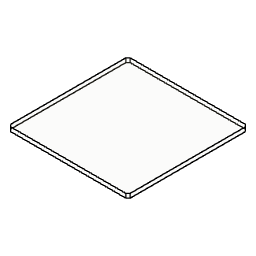
Generic Single Pad Assembly v8 (Autodesk Fusion 360 archive; units mm, degrees)
design "Polycarbonate Top"
Autodesk Fusion 360 part; units mm, degrees
sketch "Sketch1" plane through (0, 0, 0) normal (0, 0, 1) x (1, 0, 0)
  line L0 (132.5, 137.5) -> (-132.5, 137.5)
  line L1 (-137.5, 132.5) -> (-137.5, -132.5)
  line L2 (-132.5, -137.5) -> (132.5, -137.5)
  line L3 (137.5, -132.5) -> (137.5, 132.5)
  line L4 (135, 135) -> (-137.5, -137.5) construction
  line L5 (-137.5, 137.5) -> (135, -135) construction
  line L6 (137.5, 132.5) -> (132.5, 137.5)
  line L7 (-137.5, -132.5) -> (-132.5, -137.5)
  line L8 (-132.5, 137.5) -> (-137.5, 132.5)
  line L9 (137.5, -132.5) -> (132.5, -137.5)
  dimension "d2" = 275
  dimension "d5" = 5
  dimension "d6" = 5
  dimension "d7" = 5
  dimension "d8" = 5
  dimension "d9" = 5
  dimension "d10" = 5
  constraint horizontal L0
  constraint perpendicular L0 L1
  constraint parallel L0 L2
  constraint parallel L1 L3
  constraint coincident L4 origin
  constraint coincident L5 origin
  constraint coincident L3.end L6.start
  constraint coincident L0.start L6.end
  constraint coincident L6 L4.start
  constraint coincident L1.end L7.start
  constraint coincident L2.start L7.end
  constraint perpendicular L4 L7
  constraint coincident L0.end L8.start
  constraint coincident L1.start L8.end
  constraint coincident L3.start L9.start
  constraint coincident L2.end L9.end
  constraint coincident L9 L5.end
  measures "d2" distance of L5.start L4.end
  measures "d5" distance of L2 L3.start
  measures "d6" distance of L3 L2.end
  measures "d7" distance of L1 L0.end
  measures "d8" distance of L0 L1.start
  measures "d9" distance of L2 L1.end
  measures "d10" distance of L1 L2.start
extrude "Extrude1" add sketch "Sketch1" along normal blind 9.525
equation "d11 = 3 / 8 * in"

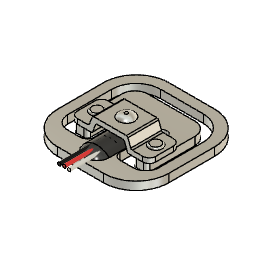
design "SparkFun Generic Load Cell"
Autodesk Fusion 360 part; units mm, degrees
sketch "Sketch1" plane through (0, 0, 0) normal (0, 0, 1) x (1, 0, 0)
  line L0 (17, -17) -> (-17, -17)
  line L1 (-17, -17) -> (-17, 17)
  line L2 (-17, 17) -> (17, 17)
  line L3 (17, 17) -> (17, -17)
  line L4 (17, -17) -> (-17, 17) construction
  line L5 (-17, -17) -> (17, 17) construction
  line L6 (-25.4453, -3) -> (28.0495, -3) construction
  line L7 (-14, 14) -> (14, 14)
  line L8 (14, 14) -> (14, -11)
  line L9 (14, -11) -> (-14, -11)
  line L10 (-14, -11) -> (-14, 14)
  line L11 (-11.2, 10.8) -> (11.2, 10.8)
  circle A0 centre (-9, -3) radius 1.5
  line L12 (0, 0) -> (0, -17) construction
  circle A1 centre (9, -3) radius 1.5
  line L13 (11.2, 10.8) -> (11.2, -8)
  line L14 (-11.2, 10.8) -> (-11.2, -8)
  line L15 (-11.2, -8) -> (11.2, -8)
  line L16 (-7, -8) -> (-7, 4)
  line L17 (7, -8) -> (7, 4)
  line L18 (-7, 4) -> (7, 4)
  line L19 (-4, 4) -> (-4, -8)
  line L20 (4, 4) -> (4, -8)
  line L21 (-4, -7.7759) -> (-4, -11)
  line L22 (4, -8) -> (4, -11)
  dimension "d1" = 34
  dimension "d2" = 34
  dimension "d3" = 14
  dimension "d4" = 3
  dimension "d5" = 3.2
  dimension "d6" = 3
  dimension "d7" = 9
  dimension "d8" = 2.8
  dimension "d9" = 6
  dimension "d10" = 3
  dimension "d11" = 7
  dimension "d12" = 21
  dimension "d13" = 4
  constraint horizontal L0
  constraint perpendicular L0 L1
  constraint parallel L0 L2
  constraint parallel L1 L3
  constraint coincident L4 L12.start
  constraint coincident L5 L12.start
  constraint coincident L12.start origin
  constraint horizontal L6
  constraint horizontal L7
  constraint vertical L8
  constraint horizontal L9
  constraint vertical L10
  constraint coincident L4 L7.start
  constraint coincident L5 L7.end
  constraint horizontal L11
  constraint coincident L6 A0.centre
  constraint midpoint L0 L12.end
  constraint symmetric A0 L12 A1
  constraint perpendicular L6 L13
  constraint symmetric L11.end L12 L11.start
  constraint symmetric L12 L13.end L14.end
  constraint coincident L15 L16.start
  constraint perpendicular L15 L16
  constraint symmetric L12 L16.start L17.start
  constraint symmetric L12 L16.end L17.end
  constraint coincident L18 L19.start
  constraint coincident L15 L19.end
  constraint perpendicular L15 L19
  constraint symmetric L12 L19.start L20.start
  constraint symmetric L12 L19.end L20.end
  constraint coincident L19 L21.start
  constraint perpendicular L9 L21
  constraint coincident L9 L21.end
  constraint coincident L9 L22.end
  constraint perpendicular L9 L22
  measures "d1" distance of L1.end L2.end
  measures "d2" distance of L0.end L1.end
  measures "d3" distance of L0 L6
  measures "d4" distance of L2 L7
  measures "d5" distance of L7 L11
  measures "d6" diameter of A0
  measures "d7" distance of A0.centre L12
  measures "d8" distance of L8 L13
  measures "d9" distance of L0 L9
  measures "d10" distance of L9 L15
  measures "d11" distance of L12 L16
  measures "d12" distance of L0 L18
  measures "d13" distance of L12 L19
extrude "Extrude1" add sketch "Sketch1" along normal blind 2.5 contours L0 L1 L2 L3 | L9 L15 L21 L22 | L15 L18 L19 L20 L21 | L11 L13 L14 L15 L16 L17 L18 makes body 1
ref_plane "WorkPlane1" through (9.1, -8, 1.25) normal (0, -1, 0) x (1, 0, 0)
sketch "Sketch2" plane through (0, -8, 0) normal (0, -1, 0) x (-1, 0, 0)
  line L0 (11.2, 0) -> (7, 0)
  line L1 (7, 0) -> (7, -2.5)
  line L2 (7, -2.5) -> (11.2, -2.5)
  line L3 (11.2, -2.5) -> (11.2, 0)
  line L4 (-7, 0) -> (-11.2, 0)
  line L5 (-11.2, 0) -> (-11.2, -2.5)
  line L6 (-11.2, -2.5) -> (-7, -2.5)
  line L7 (-7, -2.5) -> (-7, 0)
  line L8 (12, -4) -> (12, -2.5)
  line L9 (5.4, -4) -> (5.4, -2.5)
  line L10 (0, 0) -> (0, -12.4742) construction
  line L11 (12, -4) -> (5.0658, -4)
  line L12 (12, -2.5) -> (5.4, -2.5)
  line L13 (0, -7) -> (5.3584, -7)
  line L14 (5.3584, -7) -> (5.3584, -5.5)
  line L15 (5.3584, -5.5) -> (0, -5.5)
  line L16 (0, -5.5) -> (0, -7)
  line L17 (5.3584, -7) -> (6.4503, -4)
  line L18 (5.4, -2.5) -> (4.3081, -5.5)
  line L19 (-5.3584, -7) -> (-6.4503, -4)
  line L20 (0, -7) -> (-5.3584, -7)
  line L21 (-5.3584, -5.5) -> (0, -5.5)
  line L22 (-5.4, -2.5) -> (-4.3081, -5.5)
  line L23 (-12, -4) -> (-5.0658, -4)
  line L24 (-12, -2.5) -> (-5.4, -2.5)
  line L25 (-12, -4) -> (-12, -2.5)
  dimension "d17" = 5.4
  dimension "d18" = 6.6
  dimension "d19" = 1.5
  dimension "d21" = 1.5
  dimension "d22" = 1.5
  dimension "d23" = 70
  dimension "d24" = 7
  constraint vertical L8
  constraint parallel L1 L9
  constraint coincident L10.start origin
  constraint vertical L10
  constraint perpendicular L8 L11
  constraint coincident L8.start L11
  constraint coincident L9.start L11
  constraint horizontal L12
  constraint coincident L1.end L12
  constraint horizontal L13
  constraint vertical L14
  constraint horizontal L15
  constraint vertical L16
  constraint coincident L10 L13.start
  constraint coincident L11 L17.end
  constraint coincident L15 L18.end
  constraint parallel L17 L18
  constraint symmetric L8.start L10 L23.start
  constraint symmetric L8.end L10 L24.start
  constraint symmetric L10 L11.end L23.end
  constraint symmetric L10 L9.end L22.start
  constraint symmetric L10 L13.start L16.end
  constraint symmetric L10 L13.end L19.start
  constraint symmetric L10 L14.end L21.start
  constraint symmetric L10 L15.end L16.start
  constraint symmetric L10 L17.end L19.end
  constraint symmetric L10 L18.end L22.end
  measures "d17" distance of L9 L10
  measures "d18" distance of L8 L9
  measures "d19" distance of L2 L11
  measures "d21" distance of L13.start L15.end
  measures "d22" distance of L17 L18
  measures "d23" angle of L12 L18
  measures "d24" distance of L10.start L13
extrude "Extrude2" add sketch "Sketch2" against normal blind 9.4 separate body contours L2 L8 L9 L11 L12 | L9 L11 L14 L15 L17 L18 | L13 L14 L15 L16 | L6 L16 L19 L20 L21 L22 L23 L24 L25 makes body 2
sketch "Sketch3" plane through (0, 0, 7) normal (0, 0, 1) x (-1, 0, 0)
  line L0 (5.3584, 8) -> (-5.3584, 8)
  line L1 (-5.3584, 8) -> (-5.3584, -1.4)
  line L2 (-5.3584, -1.4) -> (5.3584, -1.4)
  line L3 (5.3584, -1.4) -> (5.3584, 8)
  line L4 (25.4453, 3) -> (-28.0495, 3) construction
  line L5 (0, 0) -> (0, 17) construction
  circle A0 centre (0, 3) radius 2.5
  point P0 (0, 3)
  dimension "d28" = 5
  constraint coincident L5 P0
  constraint coincident L4 P0
  constraint coincident P0 A0.centre
  measures "d28" diameter of A0
ref_plane "WorkPlane2" through (0, -3.3, 7) normal (0, 0, 1) x (1, 0, 0)
extrude "Extrude3" add sketch "Sketch3" along normal blind 1 contours A0 bodies 2
fillet "Fillet1" radius 2.5 1 edges at (2.3308, -2.096, 8) on bodies 2
fillet "Fillet2" radius 10 4 edges at (-17, 17, 1.25) (-17, -17, 1.25) (17, 17, 1.25) (17, -17, 1.25) on bodies 1
fillet "Fillet2" radius 7.5 2 edges at (-14, 14, 1.25) (14, 14, 1.25) on bodies 1
fillet "Fillet2" radius 4 2 edges at (14, -11, 1.25) (-14, -11, 1.25) on bodies 1
fillet "Fillet2" radius 2 2 edges at (4, -11, 1.25) (-4, -11, 1.25) on bodies 1
fillet "Fillet2" radius 1.5 4 edges at (-4, 4, 1.25) (-7, 4, 1.25) (4, 4, 1.25) (7, 4, 1.25) on bodies 1
fillet "Fillet2" radius 1 4 edges at (-11.2, -8, 1.25) (-7, -8, 1.25) (7, -8, 1.25) (11.2, -8, 1.25) on bodies 1
fillet "Fillet2" radius 4 2 edges at (-11.2, 10.8, 1.25) (11.2, 10.8, 1.25) on bodies 1
fillet "Fillet3" radius 2 4 edges at (-12, -8, 3.25) (12, -8, 3.25) (-12, 1.4, 3.25) (12, 1.4, 3.25) on bodies 2
fillet "Fillet3" radius 0.5 8 edges at (6.4503, -3.3, 4) (5.3584, -3.3, 7) (-5.3584, -3.3, 7) (-6.4503, -3.3, 4) (-5.4, -3.3, 2.5) (-4.3081, -3.3, 5.5) (4.3081, -3.3, 5.5) (5.4, -3.3, 2.5) on bodies 2
sketch "Sketch5" plane through (0, 0, 2.5) normal (0, 0, 1) x (-1, 0, 0)
  arc A0 (-17, -7) -> (-7, -17) centre (-7, -7) ccw
  line L0 (-7, -17) -> (7, -17)
  arc A1 (7, -17) -> (17, -7) centre (7, -7) ccw
  line L1 (17, -7) -> (17, 7)
  arc A2 (17, 7) -> (7, 17) centre (7, 7) ccw
  line L2 (7, 17) -> (-7, 17)
  arc A3 (-7, 17) -> (-17, 7) centre (-7, 7) ccw
  line L3 (-17, 7) -> (-17, -7)
  arc A4 (-11.2, -6.8) -> (-7.2, -10.8) centre (-7.2, -6.8) ccw
  line L4 (-7.2, -10.8) -> (7.2, -10.8)
  arc A5 (7.2, -10.8) -> (11.2, -6.8) centre (7.2, -6.8) ccw
  line L5 (11.2, -6.8) -> (11.2, 7)
  arc A6 (11.2, 7) -> (10.2, 8) centre (10.2, 7) ccw
  line L6 (10.2, 8) -> (8, 8)
  arc A7 (8, 8) -> (7, 7) centre (8, 7) ccw
  line L7 (7, 7) -> (7, -2.5)
  arc A8 (4, -2.5) -> (7, -2.5) centre (5.5, -2.5) ccw
  line L8 (4, -2.5) -> (4, 9)
  arc A9 (6, 11) -> (4, 9) centre (6, 9) ccw
  line L9 (6, 11) -> (10, 11)
  arc A10 (14, 7) -> (10, 11) centre (10, 7) ccw
  line L10 (14, 7) -> (14, -6.5)
  arc A11 (6.5, -14) -> (14, -6.5) centre (6.5, -6.5) ccw
  line L11 (6.5, -14) -> (-6.5, -14)
  arc A12 (-14, -6.5) -> (-6.5, -14) centre (-6.5, -6.5) ccw
  line L12 (-14, -6.5) -> (-14, 7)
  arc A13 (-10, 11) -> (-14, 7) centre (-10, 7) ccw
  line L13 (-10, 11) -> (-6, 11)
  arc A14 (-4, 9) -> (-6, 11) centre (-6, 9) ccw
  line L14 (-4, 9) -> (-4, -2.5)
  arc A15 (-7, -2.5) -> (-4, -2.5) centre (-5.5, -2.5) ccw
  line L15 (-7, -2.5) -> (-7, 7)
  arc A16 (-7, 7) -> (-8, 8) centre (-8, 7) ccw
  line L16 (-8, 8) -> (-10.2, 8)
  arc A17 (-10.2, 8) -> (-11.2, 7) centre (-10.2, 7) ccw
  line L17 (-11.2, 7) -> (-11.2, -6.8)
  circle A18 centre (-9, 3) radius 1.5
  circle A19 centre (9, 3) radius 1.5
  line L18 (0, 0) -> (0, 20.056) construction
  line L19 (0, 0) -> (0, -17) construction
  line L20 (3.75, -1.8) -> (3.75, 12)
  arc A20 (3.75, 12) -> (-3.75, 12) centre (0, 12) ccw
  line L21 (-3.75, 12) -> (-3.75, -1.8)
  arc A21 (-3.75, -1.8) -> (3.75, -1.8) centre (0, -1.8) ccw
  line L22 (0, -1.8) -> (0, 12) construction
  dimension "d52" = 7.5
  dimension "d53" = 5
  dimension "d54" = 9
  constraint coincident L18.start L19.start
  constraint perpendicular L2 L18
  constraint midpoint L0 L19.end
  constraint tangent L20 A20
  constraint tangent A20 L21
  constraint parallel L20 L21
  constraint tangent L21 A21
  constraint tangent L20 A21
  constraint coincident L18 A20.centre
  constraint parallel L18 L22
  measures "d52" diameter of A20
  measures "d53" distance of L2 A20.centre
  measures "d54" distance of L4 A21.centre
extrude "Extrude4" add sketch "Sketch5" along normal blind 1.5 separate body contours L20 A20 L21 A21 makes body 3
fillet "Fillet4" radius 5.4375 4 edges at (3.75, -5.1, 4) (0, 5.55, 4) (-3.75, -5.1, 4) (0, -15.75, 4) on bodies 3
ref_plane "WorkPlane3" through (-9.1, -8, 1.25) normal (0, -1, 0) x (1, 0, 0)
sketch "Sketch6" plane through (0, -8, 0) normal (0, -1, 0) x (-1, 0, 0)
  line L0 (0, 0) -> (0, -3.15) construction
  circle A0 centre (0, -3.15) radius 0.5
  line L1 (0, -3.15) -> (-4.0161, -3.2928) construction
  circle A1 centre (-1.5, -3.2033) radius 0.5
  circle A2 centre (1.5, -3.2033) radius 0.5
  dimension "d60" = 1
  dimension "d61" = 3.15
  dimension "d62" = 1.5
  constraint coincident L0.start origin
  constraint vertical L0
  constraint coincident L0.end A0.centre
  constraint coincident L1 A1.centre
  constraint equal A0 A1
  constraint symmetric L0 A1 A2
  measures "d60" diameter of A0
  measures "d61" distance of L0.start L0.end
  measures "d62" horizontal distance of L0.end A2.centre
extrude "Extrude5" add sketch "Sketch6" along normal blind 14 separate body makes body 4 at (-1.9975, -17.3333, 3.2531) makes body 5 at (-0.4975, -17.3333, 3.1998) makes body 6 at (1.0025, -17.3333, 3.2531)
move_body "Move1" bodies 5 to x (1, 0, 0) y (0, 1, 0) z (0, 0, 1) at (0, 0, 0)
extrude "Extrude6" cut sketch "Sketch1" along normal blind 8 contours A0 | A1 bodies 2
sketch "Sketch7" plane through (0, 0, 0) normal (0, 0, 1) x (1, 0, 0)
  circle A0 centre (-9, -3) radius 1.5
  circle A1 centre (-9, -3) radius 2
  dimension "d67" = 0.5
  constraint concentric A0 A1
  measures "d67" distance of A0 A1
extrude "Extrude7" add sketch "Sketch7" along normal blind 4 separate body contours A0 makes body 7
extrude "Extrude8" add sketch "Sketch7" against normal blind 0.5 contours A0 | A1 bodies 7
extrude "Extrude9" add sketch "Sketch7" along normal blind 0.5 from surface at 4 contours A0 | A1 bodies 7
fillet "Fillet5" radius 0.5 1 edges at (-10.8647, -3.7232, 4.5) on bodies 7
fillet "Fillet5" radius 0.5 1 edges at (-10.8647, -2.2768, -0.5) on bodies 7
mirror "Mirror1" about plane through (0, 0, 0) normal (1, 0, 0) of bodies 7 makes body 8
named bodies: "Main", "Bracket", "Resin", "Black Wire", "Red Wire", "White Wire", "Rivet 1", "Rivet 2"
